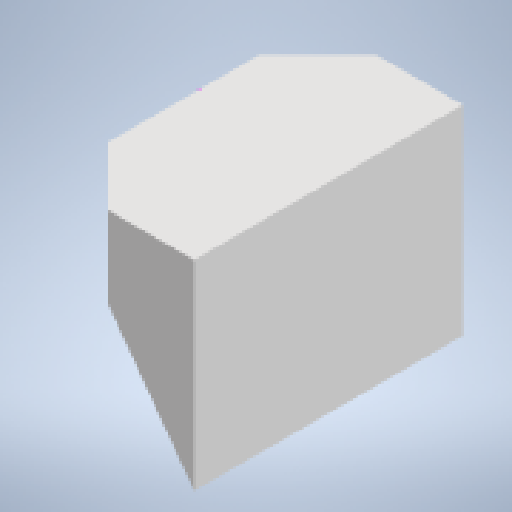
# Autodesk Inventor part: Rampa2
Saved by Autodesk Inventor 2023 (Build 270158000, 158)
## iProperties
Created: 2022-12-03
Part Number: Rampa2
Material: Genérico
Document SubType Name: Modeling
Designer: sergi
Density: 1 g/cm^3
Appearance: Valor por defecto
Author: sergi
Autodesk Inventor part; units mm, degrees
ref_plane "YZ Plane" through (0, 0, 0) normal (1, 0, 0) x (0, 1, 0)
ref_plane "XZ Plane" through (0, 0, 0) normal (0, 1, 0) x (-1, 0, 0)
ref_plane "XY Plane" through (0, 0, 0) normal (0, 0, 1) x (1, 0, 0)
sketch "Boceto1" plane through (0, 0, 0) normal (0, 1, 0) x (-1, 0, 0)
  line L0 (-18.96, -20.37) -> (-32, -20.37)
  line L1 (-32, -20.37) -> (-32, 20.37)
  line L2 (-32, 20.37) -> (-18.96, 20.37)
  line L3 (-18.96, 20.37) -> (-10, 11.41)
  line L4 (-18.96, -20.37) -> (-10, -11.41)
  line L5 (-10, 0) -> (-10, 14.0554)
  line L6 (-10, 0) -> (4.0554, 0) construction
  line L7 (-10, 14.0554) -> (-10, -14.0554)
  dimension "d15" = 13.04
  dimension "d16" = 40.74
  dimension "d17" = 13.04
  dimension "d108" = 90
  constraints: 16 end point, 4 perpendicular, 3 point on line, 2 horizontal, 1 midpoint
  measures "d15" distance of L0.start L0.end
  measures "d16" distance of L0.end L1.end
  measures "d17" distance of L1.end L2.end
  measures "d108" angle of L6 L5
extrude "Extrusión1" add sketch "Boceto1" along normal blind 20.31
sketch "Boceto7" plane through (0, 20.31, 0) normal (0, 1, 0) x (1, 0, 0)
  line L0 (6.8202, -5.4018) -> (6.8202, 5.4018) projected
  line L1 (32, -20.37) -> (32, 20.37) projected
  line L2 (32, 20.37) -> (18.96, 20.37) projected
  line L3 (18.96, 20.37) -> (10, 11.41) projected
  line L4 (10, -11.41) -> (18.96, -20.37) projected
  line L5 (18.96, -20.37) -> (32, -20.37) projected
  line L6 (10, 11.41) -> (10, -11.41) projected
  point P0 (0, 0)
extrude "Extrusión5" add sketch "Boceto7" along normal blind 10
chamfer "Chaflán2" distance 30.31 distance2 22 1 edges at (10, 0, 0) measured on face at (10, 10.1033, -3.8033)
shell "Vaciado2" thickness 2 removed faces 3 at (24.6667, 30.31, 3.8033) at (32, 0, 6.79) at (32, 10.1033, 6.79)
chamfer "Chaflán3" distance 2 angle 45 1 edges at (12.4712, 30.31, 0)
fillet "Empalme2" radius 4 1 edges at (13.646, 28.6914, 0)
sketch "Boceto13" plane through (18.96, 30.31, 20.37) normal (0, 0, 1) x (1, 0, 0)
  line L0 (13.04, 0) -> (3.04, 0)
  line L1 (3.04, 0) -> (3.04, -2)
  line L2 (3.04, -2) -> (13.04, -2)
  line L3 (13.04, -2) -> (13.04, 0)
  line L4 (13.04, 0) -> (11.04, 0)
  line L5 (11.04, 0) -> (11.04, -10)
  line L6 (11.04, -10) -> (13.04, -10)
  line L7 (13.04, -10) -> (13.04, 0)
  point P0 (-18.96, -30.31)
  point P1 (11.04, -2)
  point P2 (13.04, -2)
  dimension "d123" = 10
  dimension "d124" = 2
  dimension "d125" = 2
  dimension "d126" = 10
  constraints: 16 end point, 4 parallel, 2 horizontal, 2 perpendicular
  measures "d123" distance of L2.end L1.end
  measures "d124" distance of L1.end L0.end
  measures "d125" distance of L6.end L5.end
  measures "d126" distance of L5.end L4.end
extrude "Extrusión9" add sketch "Boceto13" along normal blind 10
sketch "Boceto14" plane through (32, 30.31, -20.37) normal (0, 0, -1) x (-1, 0, 0)
  line L0 (0, -26.9052) -> (0, 0) projected
  line L1 (0, 0) -> (10, 0)
  line L2 (10, 0) -> (10, -2)
  line L3 (10, -2) -> (0, -2)
  line L4 (0, -2) -> (0, 0)
  line L5 (0, 0) -> (12.2116, 0) projected
  line L6 (0, 0) -> (2, 0)
  line L7 (2, 0) -> (2, -10)
  line L8 (2, -10) -> (0, -10)
  line L9 (0, -10) -> (0, 0)
  point P0 (32, -30.31)
  point P1 (2, -2)
  dimension "d129" = 10
  dimension "d130" = 2
  dimension "d131" = 2
  dimension "d132" = 10
  constraints: 16 end point, 4 parallel, 2 horizontal, 2 perpendicular
  measures "d129" distance of L2.end L3.end
  measures "d130" distance of L1.end L2.end
  measures "d131" distance of L7.end L8.end
  measures "d132" distance of L6.end L7.end
extrude "Extrusión10" add sketch "Boceto14" along normal blind 10
sketch "Boceto15" plane through (32, 0, 20.37) normal (1, 0, 0) x (0, 0, -1)
  line L0 (2, 30.31) -> (-10, 30.31) projected
  line L1 (-10, 20.31) -> (-10, 30.31) projected
  line L2 (38.74, 30.31) -> (50.74, 30.31) projected
  line L3 (50.74, 30.31) -> (50.74, 20.31) projected
  point P0 (20.37, 0)
  point P1 (-5, 25.31)
  point P2 (45.74, 25.31)
  dimension "d135" = 5
  dimension "d136" = 5
  dimension "d144" = 5
  dimension "d145" = 5
  measures "d135" distance from line of L0 point (-5, 25.31)
  measures "d136" distance from line of L1 point (-5, 25.31)
  measures "d144" distance from line of L2 point (45.74, 25.31)
  measures "d145" distance from line of L3 point (45.74, 25.31)
hole "Agujero5" at (32, 25.31, 25.37) at (32, 25.31, -25.37) direction (-1, 0, 0) diameter 2 depth 2.5 tip angle 118
sketch "Boceto16" plane through (0, 30.31, 0) normal (0, 1, 0) x (1, 0, 0)
  line L0 (32, -30.37) -> (22, -30.37) projected
  line L1 (22, -20.37) -> (22, -30.37) projected
  line L2 (22, 30.37) -> (32, 30.37) projected
  line L3 (22, 20.37) -> (22, 30.37) projected
  point P0 (0, 0)
  point P1 (27, -25.37)
  point P2 (27, 25.37)
  dimension "d146" = 5
  dimension "d147" = 5
  dimension "d148" = 5
  dimension "d149" = 5
  measures "d146" distance from line of L0 point (27, -25.37)
  measures "d147" distance from line of L1 point (27, -25.37)
  measures "d148" distance from line of L2 point (27, 25.37)
  measures "d149" distance from line of L3 point (27, 25.37)
hole "Agujero6" at (27, 30.31, 25.37) at (27, 30.31, -25.37) direction (0, -1, 0) diameter 2 depth 2.5 tip angle 118
